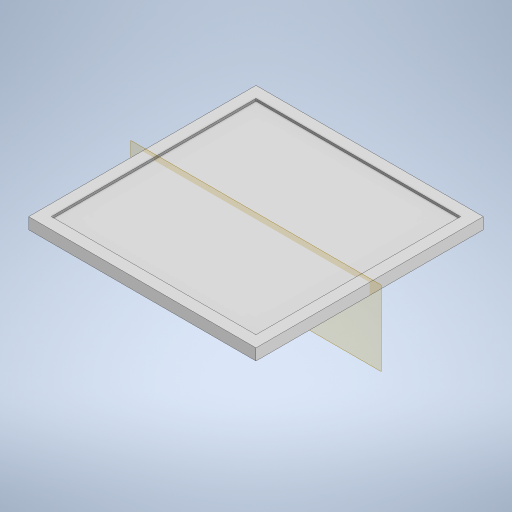
# Autodesk Inventor part: Part2
Saved by Autodesk Inventor 2023 (Build 270158000, 158)
## iProperties
Created: 2022-10-04
Part Number: Part2
Material: Generic
Document SubType Name: Modeling
Designer: Ty Gazaway
Density: 1 g/cm^3
Appearance: Default
Author: Ty Gazaway
Autodesk Inventor part; units mm, degrees
ref_plane "YZ Plane" through (0, 0, 0) normal (1, 0, 0) x (0, 1, 0)
ref_plane "XZ Plane" through (0, 0, 0) normal (0, 1, 0) x (-1, 0, 0)
ref_plane "XY Plane" through (0, 0, 0) normal (0, 0, 1) x (1, 0, 0)
sketch "Sketch1" plane through (0, 0, 0) normal (0, 1, 0) x (-1, 0, 0)
  line L0 (0, 0) -> (25.4, 0)
  line L1 (25.4, 0) -> (25.4, -25.4)
  line L2 (25.4, -25.4) -> (0, -25.4)
  line L3 (0, -25.4) -> (0, 0)
  dimension "d0" = 25.4
  dimension "d1" = 25.4
  constraints: 8 end point, 2 parallel, 1 horizontal, 1 perpendicular
  measures "d0" distance of L1.end L2.end
  measures "d1" distance of L0.end L1.end
extrude "Extrusion1" add sketch "Sketch1" along normal blind 1.27
sketch "Sketch2" plane through (0, 0, 0) normal (0, -1, 0) x (1, 0, 0)
  line L0 (-6.6675, -6.6675) -> (-18.7325, -6.6675)
  line L1 (-18.7325, -6.6675) -> (-18.7325, -18.7325)
  line L2 (-18.7325, -18.7325) -> (-6.6675, -18.7325)
  line L3 (-6.6675, -18.7325) -> (-6.6675, -6.6675)
  line L4 (0, 0) -> (0, -25.4) projected
  line L5 (0, -25.4) -> (-25.4, -25.4) projected
  line L6 (-7.9375, -7.9375) -> (-17.4625, -7.9375)
  line L7 (-17.4625, -7.9375) -> (-17.4625, -17.4625)
  line L8 (-17.4625, -17.4625) -> (-7.9375, -17.4625)
  line L9 (-7.9375, -17.4625) -> (-7.9375, -7.9375)
  point P0 (-6.6675, -12.7)
  point P1 (0, -12.7)
  point P2 (-12.7, -18.7325)
  point P3 (-12.7, -25.4)
  dimension "d4" = 12.065
  dimension "d6" = 1.27
  constraints: 16 end point, 4 midpoint, 4 parallel, 3 perpendicular, 1 horizontal, 1 horizontal alignment, 1 vertical alignment, 3 other
  measures "d4" distance of L2.end L1.end
  measures "d6" distance between parallel lines of L3 L9
extrude "Extrusion2" add sketch "Sketch2" along normal blind 6.35
sketch "Sketch3" plane through (-18.7325, 0, -6.6675) normal (0, 0, 1) x (1, 0, 0)
  line L0 (3.175, -2.54) -> (8.89, -2.54)
  line L1 (8.89, -2.54) -> (8.89, -2.794)
  line L2 (8.89, -2.794) -> (3.175, -2.794)
  line L3 (3.175, -2.794) -> (3.175, -2.54)
  line L4 (12.065, -6.35) -> (0, -6.35) projected
  line L5 (-6.6675, 0) -> (18.7325, 0) projected
  line L6 (3.175, -0.889) -> (3.429, -0.889)
  line L7 (3.429, -0.889) -> (3.429, -2.794)
  line L8 (3.429, -2.794) -> (3.175, -2.794)
  line L9 (3.175, -2.794) -> (3.175, -0.889)
  line L10 (6.0325, -2.794) -> (6.0325, -2.54) construction
  line L11 (8.89, -0.889) -> (8.636, -0.889)
  line L12 (8.636, -0.889) -> (8.636, -2.794)
  line L13 (8.89, -2.794) -> (8.89, -0.889)
  point P0 (6.0325, -6.35)
  point P1 (8.636, -2.54)
  point P2 (3.429, -2.54)
  dimension "d9" = 0.254
  dimension "d10" = 5.715
  dimension "d11" = 2.54
  dimension "d14" = 0.254
  dimension "d15" = 1.905
  constraints: 24 end point, 4 parallel, 4 symmetric about line, 3 midpoint, 2 horizontal, 2 perpendicular, 1 horizontal alignment, 1 vertical alignment
  measures "d9" distance of L0.end L1.end
  measures "d10" distance of L0.start L0.end
  measures "d11" distance between parallel lines of L5 L0
  measures "d14" distance of L7.end L8.end
  measures "d15" distance of L6.end L7.end
extrude "Extrusion3" cut sketch "Sketch3" against normal through all
chamfer "Chamfer1" distance 0.508 angle 15 1 edges at (-12.7, -2.54, -6.6675) measured on face at (-13.6525, -5.1647, -6.6675)
sketch "Sketch4" plane through (-10.0965, -2.54, -7.9375) normal (1, 0, 0) x (0, 0, -1)
  line L0 (-1.27, 0.508) -> (-1.1339, 0) projected
  line L1 (-1.27, 0.508) -> (-1.27, 1.27)
  line L2 (-1.27, 0.508) -> (-1.4742, 1.27)
  line L3 (-1.4742, 1.27) -> (-1.27, 1.27)
  line L4 (-1.27, 1.651) -> (0, 1.651) construction
  line L5 (-1.27, 1.651) -> (-1.27, 1.27) construction
  line L6 (-1.27, 0.508) -> (-1.27, 1.651) construction
  point P0 (-7.9375, 2.54)
  dimension "d22" = 0.381
  constraints: 8 end point, 2 collinear, 1 horizontal
  measures "d22" distance of L4.start L1.end
extrude "Extrusion4" add sketch "Sketch4" against normal up to surface (5.207 mm away)
ref_plane "Work Plane1" through (-18.7325, 0, -12.7) normal (0, 0, 1) x (1, 0, 0)
chamfer "Chamfer2" distance 0.508 angle 15 1 edges at (-12.7, -2.54, -18.7325) measured on face at (-11.7475, -5.1647, -18.7325)
mirror "Mirror2" about plane through (-18.7325, 0, -12.7) normal (0, 0, 1) of "Extrusion4"
sketch "Sketch5" plane through (0, 1.27, 0) normal (0, 1, 0) x (1, 0, 0)
  line L0 (0, 25.4) -> (-25.4, 25.4) projected
  line L1 (-25.4, 25.4) -> (-25.4, 0) projected
  line L2 (-25.4, 0) -> (0, 0) projected
  line L3 (0, 0) -> (0, 25.4) projected
  line L4 (-24.13, 1.27) -> (-24.13, 24.13)
  line L5 (-24.13, 24.13) -> (-1.27, 24.13)
  line L6 (-1.27, 24.13) -> (-1.27, 1.27)
  line L7 (-1.27, 1.27) -> (-24.13, 1.27)
  dimension "d26" = 1.27
  constraints: 8 end point, 3 other
  measures "d26" distance between parallel lines of L1 L4
extrude "Extrusion5" cut sketch "Sketch5" against normal blind 0.254 contours L4 L5 L6 L7
body "Solid1"
